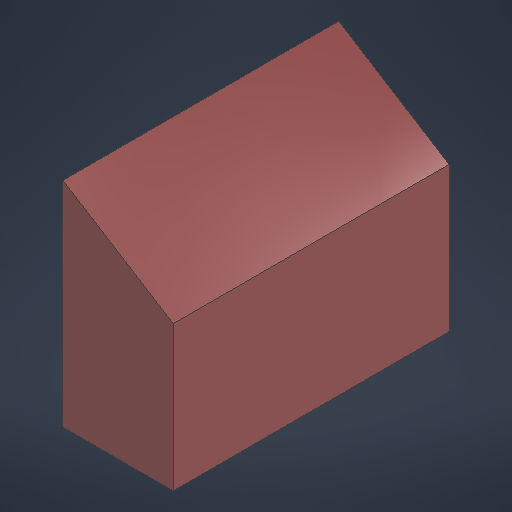
# Autodesk Inventor part: Housing og Buttons & LCD
Saved by Autodesk Inventor 2026.2 (Build 302298010, 298A)
## iProperties
Created: 2026-05-24
Part Number: Housing og Buttons & LCD
Material: Generic
Document SubType Name: Modeling
Designer: lenovo
Density: 1 g/cm^3
Appearance: Default
Author: lenovo
Autodesk Inventor part; units mm, degrees
ref_plane "YZ Plane" through (0, 0, 0) normal (1, 0, 0) x (0, 1, 0)
ref_plane "XZ Plane" through (0, 0, 0) normal (0, 1, 0) x (-1, 0, 0)
ref_plane "XY Plane" through (0, 0, 0) normal (0, 0, 1) x (1, 0, 0)
sketch "Sketch1" plane through (0, 0, 0) normal (0, 0, 1) x (1, 0, 0)
  line L0 (0, 0) -> (80, 0)
  line L1 (0, 0) -> (0, 155)
  line L2 (80, 0) -> (80, 105)
  line L3 (80, 105) -> (0, 155)
  dimension "d0" = 80
  dimension "d1" = 155
  dimension "d2" = 105
  constraints: 8 end point, 1 horizontal, 1 parallel, 1 perpendicular
  measures "d0" distance of L0.start L0.end
  measures "d1" distance of L0.start L1.end
  measures "d2" distance of L0.end L2.end
extrude "Extrusion1" add sketch "Sketch1" along normal blind 200
sketch "Sketch3" plane through (0, 0, 200) normal (0, 0, 1) x (1, 0, 0)
  line L0 (2, 0) -> (2, 151.3915)
  line L1 (80, 0) -> (80, 105) projected
  line L2 (78, 0) -> (78, 103.8915)
  line L3 (80, 105) -> (0, 155) projected
  line L4 (2, 151.3915) -> (78, 103.8915)
  line L5 (0, 0) -> (80, 0) projected
  line L6 (2, 0) -> (78, 0)
  line L7 (0, 155) -> (0, 0) projected
  dimension "d23" = 2
  dimension "d24" = 2
  dimension "d25" = 2
  constraints: 8 end point, 2 point on line, 1 parallel, 1 vertical
  measures "d23" distance between parallel lines of L3 L4
  measures "d24" distance between parallel lines of L7 L0
  measures "d25" distance between parallel lines of L1 L2
extrude "Extrusion3" cut sketch "Sketch3" against normal blind 197 contours L0 L4 L2 L5
extrude "Extrusion4" add sketch "Sketch3" against normal blind 3 contours L0 L4 L2 L5
sketch "Sketch4" plane through (0, 0, 0) normal (-1, 0, 0) x (0, 0, 1)
  line L0 (0, 155) -> (0, 0) projected
  line L1 (0, 155) -> (0, 105)
  line L2 (30, 98.8915) -> (44, 98.8915)
  line L3 (44, 98.8915) -> (44, 104.1915)
  line L4 (44, 104.1915) -> (30, 104.1915)
  line L5 (30, 104.1915) -> (30, 98.8915)
  line L6 (47, 107.1915) -> (47, 95.8915)
  line L7 (27, 100.8915) -> (27, 107.1915)
  line L8 (30, 98.8915) -> (44, 98.8915)
  line L9 (0, 155) -> (0, 105)
  line L10 (0, 155) -> (200, 155) projected
  line L11 (27, 100.8915) -> (27, 155)
  line L12 (27, 155) -> (27, 100.8915)
  line L13 (30, 98.8915) -> (44, 98.8915)
  line L14 (47, 107.1915) -> (27, 107.1915)
  dimension "d38" = 3
  dimension "d39" = 5.3
  dimension "d40" = 47.8085
  dimension "d41" = 3
  constraints: 26 end point, 4 perpendicular, 2 collinear, 2 point on line
  measures "d38" distance between parallel lines of L6 L3
  measures "d39" distance between parallel lines of L2 L4
  measures "d40" distance of L11.end L7.end
  measures "d41" distance between parallel lines of L4 L14
extrude "Extrusion5" cut sketch "Sketch4" against normal blind 10
sketch "Sketch5" plane through (2, 0, 3) normal (1, 0, 0) x (0, 0, -1)
  line L0 (-27, 98.8915) -> (-41, 98.8915) projected
  line L1 (-27, 98.8915) -> (-24, 98.8915)
  line L2 (-41, 98.8915) -> (-44, 98.8915)
  line L3 (-44, 98.8915) -> (-24, 98.8915)
  line L4 (-24, 98.8915) -> (-24, 95.8915)
  line L5 (-24, 95.8915) -> (-44, 95.8915)
  line L6 (-44, 95.8915) -> (-44, 98.8915)
  point P0 (3, 0)
  dimension "d42" = 3
  dimension "d43" = 3
  dimension "d44" = 3
  constraints: 12 end point, 3 perpendicular, 2 horizontal, 1 collinear
  measures "d42" distance of L0.start L1.end
  measures "d43" distance of L0.end L2.end
  measures "d44" distance of L1.end L4.end
extrude "Extrusion6" add sketch "Sketch5" along normal blind 60
body "Solid1"
